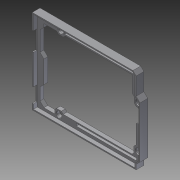
# Autodesk Inventor part: Arduino Bumper 0006
Saved by Autodesk Inventor 2012 SP1 (Build 160190100, 190)
## iProperties
Created: 2012-06-29
Part Number: Arduino Bumper 0006
Material: Default
Document SubType Name: Modeling
Designer: Chu
Density: 1 g/cm^3
Author: Chu
Autodesk Inventor part; units mm, degrees
ref_plane "YZ Plane" through (0, 0, 0) normal (1, 0, 0) x (0, 1, 0)
ref_plane "XZ Plane" through (0, 0, 0) normal (0, 1, 0) x (-1, 0, 0)
ref_plane "XY Plane" through (0, 0, 0) normal (0, 0, 1) x (1, 0, 0)
sketch "Sketch1" plane through (0, 0, 0) normal (0, 0, 1) x (1, 0, 0)
  line L0 (0, 53.34) -> (64.516, 53.34)
  line L1 (64.516, 53.34) -> (66.04, 51.816)
  line L2 (66.04, 51.816) -> (66.04, 40.386)
  line L3 (66.04, 40.386) -> (68.58, 37.846)
  line L4 (68.58, 37.846) -> (68.58, 5.08)
  line L5 (66.04, 0) -> (0, 0)
  line L6 (0, 0) -> (0, 53.34)
  line L7 (68.58, 5.08) -> (66.04, 2.54)
  line L8 (66.04, 2.54) -> (66.04, 0)
  line L9 (64.9053, 54.2798) -> (-0.9398, 54.2798)
  line L10 (-0.9398, 54.2798) -> (-0.9398, -0.9398)
  line L11 (-0.9398, -0.9398) -> (66.9798, -0.9398)
  line L12 (66.9798, -0.9398) -> (66.9798, 2.1507)
  line L13 (66.9798, 2.1507) -> (69.5198, 4.6907)
  line L14 (69.5198, 4.6907) -> (69.5198, 38.2353)
  line L15 (69.5198, 38.2353) -> (66.9798, 40.7753)
  line L16 (66.9798, 40.7753) -> (66.9798, 52.2053)
  line L17 (66.9798, 52.2053) -> (64.9053, 54.2798)
  line L18 (64.6002, 53.5432) -> (-0.2032, 53.5432)
  line L19 (-0.2032, 53.5432) -> (-0.2032, -0.2032)
  line L20 (-0.2032, -0.2032) -> (66.2432, -0.2032)
  line L21 (66.2432, -0.2032) -> (66.2432, 2.4558)
  line L22 (66.2432, 2.4558) -> (68.7832, 4.9958)
  line L23 (68.7832, 4.9958) -> (68.7832, 37.9302)
  line L24 (68.7832, 37.9302) -> (66.2432, 40.4702)
  line L25 (66.2432, 40.4702) -> (66.2432, 51.9002)
  line L26 (66.2432, 51.9002) -> (64.6002, 53.5432)
  point P0 (0, 0)
  dimension "d0" = 64.516
  dimension "d1" = 53.34
  dimension "d4" = 66.04
  dimension "d5" = 51.816
  dimension "d6" = 68.58
  dimension "d7" = 40.386
  dimension "d8" = 37.846
  dimension "d9" = 66.04
  dimension "d10" = 2.54
  dimension "d11" = 5.08
  dimension "d15" = 0.2032
  dimension "d18" = 0.7366
  constraints: 54 end point, 9 perpendicular, 6 parallel, 1 horizontal, 16 other
  measures "d0" distance of L0.start L0.end
  measures "d1" distance of L5.end L0.start
  measures "d4" distance between parallel lines of L6 L2
  measures "d5" distance from line of L5 L1.end
  measures "d6" distance between parallel lines of L6 L4
  measures "d7" distance from line of L5 L2.end
  measures "d8" distance from line of L5 L3.end
  measures "d9" distance of L5.start L5.end
  measures "d10" distance of L7.end L5.start
  measures "d11" distance from line of L5 L4.end
  measures "d15" distance between parallel lines of L18 L0
  measures "d18" distance between parallel lines of L18 L9
extrude "Extrusion2" add sketch "Sketch1" along normal blind 2.54 contours L17 L16 L15 L14 L13 L12 L11 L10 L9
sketch "Sketch2" plane through (0, 0, 0) normal (0, 0, 1) x (1, 0, 0)
  line L0 (0, 53.34) -> (64.516, 53.34)
  line L1 (64.516, 53.34) -> (66.04, 51.816)
  line L2 (66.04, 51.816) -> (66.04, 40.386)
  line L3 (66.04, 40.386) -> (68.58, 37.846)
  line L4 (68.58, 37.846) -> (68.58, 5.08)
  line L5 (66.04, 0) -> (0, 0)
  line L6 (0, 0) -> (0, 53.34)
  line L7 (68.58, 5.08) -> (66.04, 2.54)
  line L8 (66.04, 2.54) -> (66.04, 0)
  line L9 (64.9053, 54.2798) -> (-0.9398, 54.2798)
  line L10 (-0.9398, 54.2798) -> (-0.9398, -0.9398)
  line L11 (-0.9398, -0.9398) -> (66.9798, -0.9398)
  line L12 (66.9798, -0.9398) -> (66.9798, 2.1507)
  line L13 (66.9798, 2.1507) -> (69.5198, 4.6907)
  line L14 (69.5198, 4.6907) -> (69.5198, 38.2353)
  line L15 (69.5198, 38.2353) -> (66.9798, 40.7753)
  line L16 (66.9798, 40.7753) -> (66.9798, 52.2053)
  line L17 (66.9798, 52.2053) -> (64.9053, 54.2798)
  line L18 (64.6002, 53.5432) -> (-0.2032, 53.5432)
  line L19 (-0.2032, 53.5432) -> (-0.2032, -0.2032)
  line L20 (-0.2032, -0.2032) -> (66.2432, -0.2032)
  line L21 (66.2432, -0.2032) -> (66.2432, 2.4558)
  line L22 (66.2432, 2.4558) -> (68.7832, 4.9958)
  line L23 (68.7832, 4.9958) -> (68.7832, 37.9302)
  line L24 (68.7832, 37.9302) -> (66.2432, 40.4702)
  line L25 (66.2432, 40.4702) -> (66.2432, 51.9002)
  line L26 (66.2432, 51.9002) -> (64.6002, 53.5432)
  line L27 (61.8998, 49.1998) -> (61.8998, 38.6711)
  line L28 (61.8998, 38.6711) -> (63.1825, 37.3884)
  line L29 (62.9793, 5.3344) -> (61.8998, 4.2549)
  line L30 (61.8998, 4.2549) -> (61.8998, 4.1402)
  line L31 (4.1402, 4.1402) -> (4.1402, 49.1998)
  line L32 (63.627, 30.43) -> (66.167, 30.43) construction
  line L33 (66.167, 30.43) -> (66.167, 25.35) construction
  line L34 (66.167, 25.35) -> (63.627, 25.35) construction
  line L35 (63.627, 25.35) -> (63.627, 30.43) construction
  circle A0 centre (15.24, 50.8) radius 1.5875
  circle A1 centre (66.04, 35.3568) radius 1.5875
  circle A2 centre (65.8368, 7.62) radius 1.5875
  circle A3 centre (13.97, 2.54) radius 1.5875
  line L36 (13.7585, 47.9425) -> (16.8275, 47.9425)
  line L37 (16.8275, 47.9425) -> (18.0848, 49.1998)
  line L38 (13.7585, 47.9425) -> (12.5012, 49.1998)
  line L39 (4.1402, 49.1998) -> (12.5012, 49.1998)
  line L40 (18.0848, 49.1998) -> (61.8998, 49.1998)
  line L41 (63.1825, 37.3884) -> (63.1825, 33.7693)
  line L42 (63.1825, 33.7693) -> (64.4398, 32.512)
  line L43 (62.9793, 9.2075) -> (62.9793, 5.3344)
  line L44 (62.9793, 9.2075) -> (64.4398, 10.668)
  line L45 (64.4398, 32.512) -> (64.4398, 10.668)
  line L46 (12.3825, 5.3344) -> (15.5575, 5.3344)
  line L47 (15.5575, 5.3344) -> (16.7517, 4.1402)
  line L48 (12.3825, 5.3344) -> (11.1883, 4.1402)
  line L49 (61.8998, 4.1402) -> (16.7517, 4.1402)
  line L50 (11.1883, 4.1402) -> (4.1402, 4.1402)
  point P0 (0, 0)
  point P1 (0, 1.4137)
  point P2 (64.4398, 6.7949)
  dimension "d19" = 64.516
  dimension "d20" = 53.34
  dimension "d21" = 66.04
  dimension "d22" = 51.816
  dimension "d23" = 68.58
  dimension "d24" = 40.386
  dimension "d25" = 37.846
  dimension "d26" = 66.04
  dimension "d27" = 2.54
  dimension "d28" = 5.08
  dimension "d29" = 0.2032
  dimension "d30" = 0.7366
  dimension "d56" = 30.43
  dimension "d57" = 63.627
  dimension "d58" = 5.08
  dimension "d61" = 2.54
  dimension "d70" = 13.97
  dimension "d71" = 2.54
  dimension "d72" = 3.175
  dimension "d73" = 50.8
  dimension "d74" = 3.175
  dimension "d75" = 15.24
  dimension "d76" = 66.04
  dimension "d77" = 35.56
  dimension "d78" = 3.175
  dimension "d79" = 3.175
  dimension "d80" = 66.04
  dimension "d81" = 7.62
  dimension "d135" = 2.54
  dimension "d136" = 1.27
  dimension "d137" = 2.8575
  dimension "d138" = 1.27
  constraints: 102 end point, 23 perpendicular, 16 parallel, 4 centre point, 2 horizontal, 16 other
  measures "d19" distance of L0.start L0.end
  measures "d20" distance of L5.end L0.start
  measures "d21" distance between parallel lines of L6 L2
  measures "d22" distance from line of L5 L1.end
  measures "d23" distance between parallel lines of L6 L4
  measures "d24" distance from line of L5 L2.end
  measures "d25" distance from line of L5 L3.end
  measures "d26" distance of L5.start L5.end
  measures "d27" distance of L7.end L5.start
  measures "d28" distance from line of L5 L4.end
  measures "d29" distance between parallel lines of L18 L0
  measures "d30" distance between parallel lines of L18 L9
  measures "d56" distance from line of point (0, 0) L32
  measures "d57" horizontal distance of point (0, 0) L32.start
  measures "d58" distance between parallel lines of L32 L34
  measures "d61" distance between parallel lines of L33 L35
  measures "d70" horizontal distance of A3.centre point (0, 1.414)
  measures "d71" vertical distance of point (0, 0) A3.centre
  measures "d72" diameter of A3
  measures "d73" vertical distance of point (0, 0) A0.centre
  measures "d74" diameter of A0
  measures "d75" horizontal distance of point (0, 0) A0.centre
  measures "d76" horizontal distance of point (0, 0) A1.centre
  measures "d77" vertical distance of L19.end A1.centre
  measures "d78" diameter of A1
  measures "d79" diameter of A2
  measures "d80" horizontal distance of L19.end A2.centre
  measures "d81" vertical distance of A2.centre point (0, 0)
  measures "d135" distance from line of L0 A0.centre
  measures "d136" distance edge to line of A0 L36
  measures "d137" distance from line of L41 A1.centre
  measures "d138" distance edge to line of A2 L43
extrude "Extrusion3" add sketch "Sketch2" against normal blind 2.54 contours L0 L1 L2 L3 L4 L7 L8 L5 L6 | L17 L16 L15 L14 L13 L12 L11 L10 L9 | L26 L25 L24 L23 L22 L21 L20 L19 L18
sketch "Sketch4" plane through (0, 0, 2.54) normal (0, 0, 1) x (1, 0, 0)
  line L0 (-0.2032, -0.2032) -> (-0.2032, 53.5432) projected
  line L1 (-0.9398, -0.9398) -> (-0.9398, 54.2798) projected
  line L2 (-0.2032, 12.446) -> (-0.9398, 12.446)
  line L3 (-0.2032, 2.8575) -> (-0.9398, 2.8575)
  line L4 (-0.2032, 32.004) -> (-0.9398, 32.004)
  line L5 (-0.2032, 44.196) -> (-0.9398, 44.196)
  point P0 (0, 0)
  dimension "d35" = 12.446
  dimension "d36" = 2.8575
  dimension "d37" = 32.004
  dimension "d38" = 44.196
  constraints: 8 end point, 8 point on line, 4 perpendicular
  measures "d35" distance from line of point (0, 0) L2
  measures "d36" distance from line of point (0, 0) L3
  measures "d37" distance from line of point (0, 0) L4
  measures "d38" distance from line of point (0, 0) L5
extrude "Extrusion4" cut sketch "Sketch4" against normal blind 2.286 contours L3 L1 L2 L0 | L4 L1 L5 L0
sketch "Sketch5" plane through (0, 0, 0) normal (0, 0, 1) x (1, 0, 0)
  line L0 (25.4, 3.3338) -> (64.77, 3.3338)
  line L1 (64.77, 3.3338) -> (64.77, 1.7463)
  line L2 (64.77, 1.7463) -> (25.4, 1.7463)
  line L3 (25.4, 1.7463) -> (25.4, 3.3338)
  line L4 (17.78, 51.5938) -> (64.77, 51.5938)
  line L5 (64.77, 51.5938) -> (64.77, 50.0062)
  line L6 (64.77, 50.0062) -> (17.78, 50.0062)
  line L7 (17.78, 50.0062) -> (17.78, 51.5938)
  line L8 (-0.2032, 53.5432) -> (-0.2032, -0.2032) projected
  line L9 (-0.2032, 12.065) -> (11.2268, 12.065)
  line L10 (11.2268, 12.065) -> (11.2268, 1.6002)
  line L11 (11.2268, 1.6002) -> (-0.2032, 1.6002)
  line L12 (-0.2032, 1.6002) -> (-0.2032, 12.065)
  line L13 (1.6002, 12.065) -> (1.6002, 1.6002)
  line L14 (63.627, 30.43) -> (66.167, 30.43) construction
  line L15 (63.627, 25.35) -> (63.627, 30.43) construction
  line L16 (66.167, 30.43) -> (66.167, 25.35) construction
  line L17 (66.167, 25.35) -> (63.627, 25.35) construction
  line L18 (4.1402, 4.1402) -> (4.1402, 49.1998) projected
  line L19 (4.1402, 49.1998) -> (12.5012, 49.1998) projected
  line L20 (61.8998, 49.1998) -> (61.8998, 38.6711) projected
  line L21 (61.8998, 38.6711) -> (63.1825, 37.3884) projected
  line L22 (64.4398, 32.512) -> (64.4398, 10.668) projected
  line L23 (62.9793, 5.3344) -> (61.8998, 4.2549) projected
  line L24 (61.8998, 4.2549) -> (61.8998, 4.1402) projected
  line L25 (61.8998, 4.1402) -> (16.7517, 4.1402) projected
  line L26 (66.2432, 51.9002) -> (64.6002, 53.5432) projected
  line L27 (64.6002, 53.5432) -> (-0.2032, 53.5432) projected
  line L28 (-0.2032, 53.5432) -> (-0.2032, -0.2032) projected
  line L29 (-0.2032, -0.2032) -> (66.2432, -0.2032) projected
  line L30 (66.2432, -0.2032) -> (66.2432, 2.4558) projected
  line L31 (66.2432, 2.4558) -> (68.7832, 4.9958) projected
  line L32 (68.7832, 4.9958) -> (68.7832, 37.9302) projected
  line L33 (68.7832, 37.9302) -> (66.2432, 40.4702) projected
  line L34 (66.2432, 40.4702) -> (66.2432, 51.9002) projected
  line L35 (64.4398, 32.512) -> (64.4398, 10.668) projected
  line L36 (64.4398, 33.732) -> (66.9798, 31.192)
  line L37 (64.4398, 22.048) -> (66.9798, 24.588)
  line L38 (66.9798, 31.192) -> (66.9798, 24.588)
  line L39 (64.4398, 33.732) -> (64.4398, 22.048)
  line L40 (61.8998, 4.1402) -> (16.7517, 4.1402) projected
  line L41 (4.1402, 4.1402) -> (4.1402, 49.1998) projected
  line L42 (1.6002, 44.4853) -> (4.1402, 47.0253)
  line L43 (66.2432, 40.4702) -> (66.2432, 51.9002) projected
  line L44 (1.6002, 31.7147) -> (4.1402, 29.1747)
  line L45 (1.6002, 31.7147) -> (1.6002, 44.4853)
  line L46 (4.1402, 47.0253) -> (4.1402, 29.1747)
  line L47 (12.5012, 49.1998) -> (13.7585, 47.9425) projected
  line L48 (13.7585, 47.9425) -> (16.8275, 47.9425) projected
  line L49 (16.8275, 47.9425) -> (18.0848, 49.1998) projected
  line L50 (18.0848, 49.1998) -> (61.8998, 49.1998) projected
  line L51 (63.1825, 37.3884) -> (63.1825, 33.7693) projected
  line L52 (63.1825, 33.7693) -> (64.4398, 32.512) projected
  line L53 (64.4398, 10.668) -> (62.9793, 9.2075) projected
  line L54 (62.9793, 9.2075) -> (62.9793, 5.3344) projected
  line L55 (11.1883, 4.1402) -> (4.1402, 4.1402) projected
  line L56 (16.7517, 4.1402) -> (15.5575, 5.3344) projected
  line L57 (15.5575, 5.3344) -> (12.3825, 5.3344) projected
  line L58 (12.3825, 5.3344) -> (11.1883, 4.1402) projected
  point P0 (0, 0)
  point P1 (64.4398, 6.7949)
  point P2 (64.4398, 36.1311)
  point P3 (64.4398, 31.192)
  point P4 (64.4398, 31.192)
  point P5 (64.4398, 24.588)
  point P6 (64.4398, 24.588)
  dimension "d41" = 1.5875
  dimension "d42" = 25.4
  dimension "d43" = 64.77
  dimension "d44" = 17.78
  dimension "d45" = 64.77
  dimension "d46" = 1.5875
  dimension "d47" = 51.5938
  dimension "d48" = 1.7463
  dimension "d51" = 0
  dimension "d52" = 12.065
  dimension "d54" = 11.43
  dimension "d66" = 2.54
  dimension "d67" = 2.54
  dimension "d68" = 2.54
  dimension "d69" = 2.54
  dimension "d97" = 2.54
  dimension "d101" = 2.54
  dimension "d102" = 2.54
  constraints: 42 end point, 8 parallel, 6 point on line, 3 horizontal, 3 perpendicular, 2 collinear
  measures "d41" distance between parallel lines of L0 L2
  measures "d42" horizontal distance of point (0, 0) L2.end
  measures "d43" horizontal distance of point (0, 0) L1.end
  measures "d44" horizontal distance of point (0, 0) L6.end
  measures "d45" horizontal distance of point (0, 0) L4.end
  measures "d46" distance between parallel lines of L4 L6
  measures "d47" distance from line of point (0, 0) L4
  measures "d48" distance from line of point (0, 0) L2
  measures "d51" distance between parallel lines of L8 L12
  measures "d52" distance from line of point (0, 0) L9
  measures "d54" distance from line of L8.end L10
  measures "d66" distance of L36.start point (64.44, 31.192)
  measures "d67" distance of L36.end point (64.44, 31.192)
  measures "d68" distance of L37.start point (64.44, 24.588)
  measures "d69" distance of L37.end point (64.44, 24.588)
  measures "d97" distance between parallel lines of L40 L11
  measures "d101" distance between parallel lines of L18 L45
  measures "d102" distance between parallel lines of L18 L13
extrude "Extrusion5" cut sketch "Sketch5" against normal blind 2.159 contours L0 L1 L2 L3 | L4 L5 L6 L7
sketch "Sketch7" plane through (0, 0, 0) normal (0, 0, 1) x (1, 0, 0)
  line L0 (25.4, 3.3338) -> (64.77, 3.3338)
  line L1 (64.77, 3.3338) -> (64.77, 1.7463)
  line L2 (64.77, 1.7463) -> (25.4, 1.7463)
  line L3 (25.4, 1.7463) -> (25.4, 3.3338)
  line L4 (17.78, 51.5938) -> (64.77, 51.5938)
  line L5 (64.77, 51.5938) -> (64.77, 50.0062)
  line L6 (64.77, 50.0062) -> (17.78, 50.0062)
  line L7 (17.78, 50.0062) -> (17.78, 51.5938)
  line L8 (-0.2032, 53.5432) -> (-0.2032, -0.2032)
  line L9 (-0.2032, 12.065) -> (11.2268, 12.065)
  line L10 (11.2268, 12.065) -> (11.2268, 1.6002)
  line L11 (11.2268, 1.6002) -> (-0.2032, 1.6002)
  line L12 (-0.2032, 1.6002) -> (-0.2032, 12.065)
  line L13 (1.6002, 12.065) -> (1.6002, 1.6002)
  line L14 (63.627, 30.43) -> (66.167, 30.43) construction
  line L15 (63.627, 25.35) -> (63.627, 30.43) construction
  line L16 (66.167, 30.43) -> (66.167, 25.35) construction
  line L17 (66.167, 25.35) -> (63.627, 25.35) construction
  line L18 (4.1402, 4.1402) -> (4.1402, 49.1998)
  line L19 (4.1402, 49.1998) -> (61.8998, 49.1998)
  line L20 (61.8998, 49.1998) -> (61.8998, 38.6711)
  line L21 (61.8998, 38.6711) -> (64.4398, 36.1311)
  line L22 (64.4398, 6.866) -> (64.4398, 6.7949)
  line L23 (64.4398, 6.7949) -> (61.8998, 4.2549)
  line L24 (61.8998, 4.2549) -> (61.8998, 4.1402)
  line L25 (61.8998, 4.1402) -> (4.1402, 4.1402)
  line L26 (66.2432, 51.9002) -> (64.6002, 53.5432)
  line L27 (64.6002, 53.5432) -> (-0.2032, 53.5432)
  line L28 (-0.2032, 53.5432) -> (-0.2032, -0.2032)
  line L29 (-0.2032, -0.2032) -> (66.2432, -0.2032)
  line L30 (66.2432, -0.2032) -> (66.2432, 2.4558)
  line L31 (66.2432, 2.4558) -> (68.7832, 4.9958)
  line L32 (68.7832, 4.9958) -> (68.7832, 37.9302)
  line L33 (68.7832, 37.9302) -> (66.2432, 40.4702)
  line L34 (66.2432, 40.4702) -> (66.2432, 51.9002)
  line L35 (64.4398, 36.1311) -> (64.4398, 6.7949)
  line L36 (65.7098, 32.462) -> (66.9798, 31.192)
  line L37 (65.7098, 23.318) -> (66.9798, 24.588)
  line L38 (66.9798, 31.192) -> (66.9798, 24.588)
  line L39 (64.4398, 33.732) -> (64.4398, 22.048)
  line L40 (61.8998, 4.1402) -> (4.1402, 4.1402)
  line L41 (4.1402, 4.1402) -> (4.1402, 49.1998)
  line L42 (1.6002, 44.4853) -> (4.1402, 47.0253)
  line L43 (66.2432, 40.4702) -> (66.2432, 51.9002)
  line L44 (1.6002, 31.7147) -> (4.1402, 29.1747)
  line L45 (1.6002, 31.7147) -> (1.6002, 44.4853)
  line L46 (4.1402, 47.0253) -> (4.1402, 29.1747)
  arc A0 (64.4398, 8.374) -> (64.4398, 6.866) centre (65.8368, 7.62) ccw
  line L47 (64.4398, 36.1311) -> (64.4398, 8.374)
  line L48 (64.4398, 32.462) -> (65.7098, 32.462)
  line L49 (65.7098, 23.318) -> (65.0748, 23.318)
  line L50 (65.0748, 23.318) -> (64.4398, 22.683)
  point P0 (0, 0)
  point P1 (0, 0)
  point P2 (64.4398, 31.192)
  point P3 (64.4398, 31.192)
  point P4 (64.4398, 24.588)
  point P5 (64.4398, 24.588)
  dimension "d106" = 1.5875
  dimension "d107" = 25.4
  dimension "d108" = 64.77
  dimension "d109" = 17.78
  dimension "d110" = 64.77
  dimension "d111" = 1.5875
  dimension "d112" = 51.5938
  dimension "d113" = 1.7463
  dimension "d114" = 0
  dimension "d115" = 12.065
  dimension "d116" = 11.43
  dimension "d117" = 2.54
  dimension "d118" = 2.54
  dimension "d119" = 2.54
  dimension "d120" = 2.54
  dimension "d121" = 2.54
  dimension "d122" = 2.54
  dimension "d123" = 2.54
  constraints: 102 end point, 8 parallel, 8 point on line, 5 perpendicular, 3 horizontal, 2 collinear, 2 point on circle, 1 centre point
  measures "d106" distance between parallel lines of L0 L2
  measures "d107" horizontal distance of point (0, 0) L2.end
  measures "d108" horizontal distance of point (0, 0) L1.end
  measures "d109" horizontal distance of point (0, 0) L6.end
  measures "d110" horizontal distance of point (0, 0) L4.end
  measures "d111" distance between parallel lines of L4 L6
  measures "d112" distance from line of point (0, 0) L4
  measures "d113" distance from line of point (0, 0) L2
  measures "d114" distance between parallel lines of L8 L12
  measures "d115" distance from line of point (0, 0) L9
  measures "d116" distance from line of L8.end L10
  measures "d117" distance of L39.start point (64.44, 31.192)
  measures "d118" distance of L36.end point (64.44, 31.192)
  measures "d119" distance of L39.end point (64.44, 24.588)
  measures "d120" distance of L37.end point (64.44, 24.588)
  measures "d121" distance between parallel lines of L40 L11
  measures "d122" distance between parallel lines of L18 L45
  measures "d123" distance between parallel lines of L18 L13
extrude "Extrusion7" cut sketch "Sketch7" against normal through all contours L9 L18 L25 L10 L11 L13 | L9 L10 L25 L18 | L44 L45 L42 L18 | L48 L36 L38 L37 L49 L50 L35
chamfer "Chamfer3" distance 2.54 angle 45 1 edges at (4.1402, 12.065, -1.27)
chamfer "Chamfer5" distance 2.54 angle 45 1 edges at (1.6002, 1.6002, -1.27)
chamfer "Chamfer6" distance 0.381 angle 45 8 edges at (64.4525, 35.3568, 0) (64.2493, 7.62, 0) (12.3825, 2.54, 0) (13.6525, 50.8, 0) (13.6525, 50.8, -2.54) (12.3825, 2.54, -2.54) (64.2493, 7.62, -2.54) (64.4525, 35.3568, -2.54)
equation "\"d67\" = d66"
equation "\"d69\" = d68"
equation "\"d97\" = d101"
equation "\"d102\" = d101"
body "Solid2"
